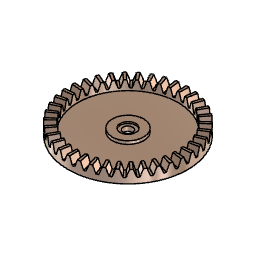
Crown Face Gear (Autodesk Fusion 360 design; units mm, degrees)
Autodesk Fusion 360 part; units mm, degrees
sketch "teeth base" plane through (0, 0, 0) normal (0, 0, 1) x (1, 0, 0)
  circle A0 centre (0, 0) radius 9.5
  circle A1 centre (0, 0) radius 8
  line L0 (0, 0) -> (14, 0) construction
  line L1 (0, 0) -> (14.107, 0.5835) construction
  line L2 (0, 0) -> (13.1414, -0.5508) construction
  dimension "d1" = 19
  dimension "d2" = 16
  dimension "d3" = 2.368
  dimension "d4" = 2.4
  constraint coincident A0.centre A1.centre
  constraint horizontal L0
  measures "d1" diameter of A0
  measures "d2" diameter of A1
  measures "d3" angle of L0 L1
  measures "d4" angle of L0 L2
ref_plane "WorkPlane1" through (9.5, 0, 0) normal (1, 0, 0) x (0, 1, 0)
sketch "loft" plane through (9.5, 0, 0) normal (1, 0, 0) x (0, 1, 0)
  line L0 (-0.5802, 0.5) -> (-0.1707, -0.625)
  line L1 (-0.1707, -0.625) -> (0.1654, -0.625)
  line L2 (0.1654, -0.625) -> (0.5749, 0.5)
  line L3 (0.5749, 0.5) -> (-0.5802, 0.5)
  line L4 (9.5, 0) -> (-9.5, 0)
  point P0 (-0.3982, 0)
  point P1 (0.3929, 0)
  dimension "d6" = 70
  dimension "d7" = 70
  dimension "d8" = 0.5
  dimension "d9" = 0.625
  constraint horizontal L1
  constraint parallel L1 L3
  constraint coincident P0 L0
  constraint coincident P1 L2
  measures "d6" angle of L2 L4
  measures "d7" angle of L0 L4
  measures "d8" distance of L3 L4
  measures "d9" distance of L1 L4
ref_plane "WorkPlane2" through (0, 0, 0.5) normal (0, 0, 1) x (1, 0, 0)
ref_plane "WorkPlane3" through (0, 0, -0.625) normal (0, 0, 1) x (1, 0, 0)
sketch "upper lines" plane through (0, 0, 0.5) normal (0, 0, 1) x (1, 0, 0)
  line L0 (0, 0) -> (9.5, 0.5749)
  line L1 (0, 0) -> (9.5, -0.5802)
  point P0 (9.5, -0.5802)
  point P1 (9.5, 0.5749)
  constraint coincident L0.start L1.start
  constraint coincident P1 L0.end
  constraint coincident P0 L1.end
sketch "bottom lines" plane through (0, 0, -0.625) normal (0, 0, 1) x (1, 0, 0)
  line L0 (0, 0) -> (9.5, -0.1707)
  line L1 (0, 0) -> (9.5, 0.1654)
  point P0 (9.5, 0.1654)
  point P1 (9.5, -0.1707)
  constraint coincident L0.start L1.start
  constraint coincident P1 L0.end
  constraint coincident P0 L1.end
ref_plane "WorkPlane4" through (7.5, 0, 0) normal (1, 0, 0) x (0, 1, 0)
sketch "cut" plane through (7.5, 0, 0) normal (1, 0, 0) x (0, 1, 0)
  line L0 (-0.458, 0.5) -> (0.4539, 0.5)
  line L1 (0.4539, 0.5) -> (0.1306, -0.625)
  line L2 (0.1306, -0.625) -> (-0.1348, -0.625)
  line L3 (-0.1348, -0.625) -> (-0.458, 0.5)
  point P0 (-0.458, 0.5)
  point P1 (0.4539, 0.5)
  point P2 (0.1306, -0.625)
  point P3 (-0.1348, -0.625)
  constraint coincident P0 L0.start
  constraint coincident P1 L0.end
  constraint coincident P2 L1.end
  constraint coincident P3 L2.end
extrude "Extrude1" add sketch "teeth base" along normal blind 0.5 and the other way blind 1 in component "Crown face gear"
loft "Loft1" cut profiles "cut", "loft" section 1 section 2 in component "Crown face gear"
pattern_circular "C-Pattern1" count 38 over 360 about axis through (0, 0, 1.75) along (0, 0, 1) of "Loft1" in component "Crown face gear"
sketch "base" plane through (0, 0, -1) normal (0, 0, -1) x (1, 0, 0)
  circle A0 centre (0, 0) radius 8
  circle A1 centre (0, 0) radius 9.5
  circle A2 centre (0, 0) radius 9.5
  dimension "d19" = 19
  constraint coincident A0.centre A1.centre
  measures "d19" diameter of A2
extrude "Extrude2" add sketch "base" along normal blind 0.5 contours A0 | A1 A2 in component "Crown face gear"
sketch "circles" plane through (0, 0, -1) normal (0, 0, 1) x (-1, 0, 0)
  circle A0 centre (0, 0) radius 8
  circle A1 centre (0, 0) radius 0.75
  circle A2 centre (0, 0) radius 1.25
  circle A3 centre (0, 0) radius 2.5
  dimension "d22" = 1.5
  dimension "d23" = 2.5
  dimension "d24" = 5
  constraint coincident A0.centre A1.centre
  constraint concentric A2 A3
  measures "d22" diameter of A1
  measures "d23" diameter of A2
  measures "d24" diameter of A3
extrude "Extrude3" cut sketch "circles" against normal blind 3 contours A1 in component "Crown face gear"
extrude "Extrude4" add sketch "circles" along normal blind 0.25 contours A2 in component "Crown face gear"
extrude "Extrude5" add sketch "circles" along normal blind 0.5 contours A3 in component "Crown face gear"
component "Crown face gear" placed x (1, 0, 0) y (0, 1, 0) z (0, 0, 1) at (0, 0, 0)
equation "d3 = ( 360 / ( 38 * 4 ) ) * 1 deg"
equation "d5 = ( 19 / 2 ) * 1 mm"
equation "d9 = ( 0.5 * 1.25 ) * 1 mm"
equation "d11 = -0.5 * 1.25 mm"
